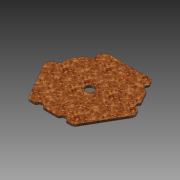
# Autodesk Inventor part: Heatbed_Insulator_Cork
Saved by Autodesk Inventor 2014 (Build 180170000, 170)
## iProperties
Created: 2014-11-03
Part Number: Heatbed_Insulator_Cork
Material: Cork Tiles
Document SubType Name: Modeling
Designer: ThatOtherGuy
Density: 0.11 g/cm^3
Appearance: Cork - Coarse
Author: ThatOtherGuy
Comments: Lowes #34744 or #33530
Autodesk Inventor part; units mm, degrees
ref_plane "YZ Plane" through (0, 0, 0) normal (1, 0, 0) x (0, 1, 0)
ref_plane "XZ Plane" through (0, 0, 0) normal (0, 1, 0) x (-1, 0, 0)
ref_plane "XY Plane" through (0, 0, 0) normal (0, 0, 1) x (1, 0, 0)
sketch "Sketch1" plane through (0, 0, 0) normal (0, 0, 1) x (1, 0, 0)
  line L0 (51.9615, 90) -> (103.923, 0)
  line L1 (103.923, 0) -> (51.9615, -90)
  line L2 (51.9615, -90) -> (-51.9615, -90)
  line L3 (-51.9615, -90) -> (-103.923, 0)
  line L4 (-103.923, 0) -> (-51.9615, 90)
  line L5 (-51.9615, 90) -> (51.9615, 90)
  circle A0 centre (0, 0) radius 10
  dimension "d3" = 180
  dimension "d13" = 20
  constraints: 12 end point, 2 coincident, 1 centre point, 1 horizontal, 13 other
  measures "d3" distance between parallel lines of L2 L5
  measures "d13" diameter of A0
extrude "Extrusion1" add sketch "Sketch1" along normal blind 4.7625
sketch "Sketch2" plane through (0, 0, 0) normal (0, 0, -1) x (-1, 0, 0)
  line L0 (-51.9615, 90) -> (-103.923, 0) projected
  line L1 (51.9615, -90) -> (103.923, 0) projected
  line L2 (103.923, 0) -> (51.9615, 90) projected
  line L3 (51.9615, 90) -> (-51.9615, 90) projected
  line L4 (-51.9615, 90) -> (0, 180) construction
  line L5 (0, 180) -> (51.9615, 90) construction
  arc A0 (-68.5, 61.3545) -> (-61, 74.3449) centre (-64.75, 67.8497) ccw
  arc A1 (-46.6506, 90) -> (-54.617, 85.4006) centre (-46.6506, 80.8013) ccw
  arc A2 (-94.8846, 15.6551) -> (-87.3846, 28.6455) centre (-91.1346, 22.1503) ccw
  line L6 (-103.923, 0) -> (-155.8846, -90) construction
  line L7 (-155.8846, -90) -> (-51.9615, -90) construction
  line L8 (-103.923, 0) -> (-51.9615, -90) projected
  arc A3 (-101.2676, 4.5994) -> (-101.2676, -4.5994) centre (-93.3013, 0) ccw
  point P0 (0, 0)
  dimension "d5" = 7.5
  dimension "d6" = 129.5
  dimension "d7" = 9.1987
  dimension "d8" = 93.3013
  dimension "d9" = 129.5
  constraints: 8 end point, 8 point on circle, 4 centre point, 2 equal radius, 2 parallel, 2 point on line, 2 tangent, 1 collinear, 12 other
  measures "d5" radius of A0
  measures "d6" distance of L4.end A0.centre
  measures "d7" radius of A1
  measures "d8" distance of point (0, 0) A1.centre
  measures "d9" distance of A2.centre L6.end
extrude "Extrusion2" cut sketch "Sketch2" against normal up to next
pattern_circular "Circular Pattern1" count 3 over 360 about axis through (0, 0, 0) along (0, 0, 1) of "Extrusion2"
fillet "Fillet1" radius 5 12 edges at (61, 74.3449, 2.3813) (68.5, 61.3545, 2.3813) (87.3846, 28.6455, 2.3813) (94.8846, 15.6551, 2.3813) (-68.5, 61.3545, 2.3813) (-61, 74.3449, 2.3813) (-94.8846, 15.6551, 2.3813) (-87.3846, 28.6455, 2.3813) (-18.8846, -90, 2.3813) (-33.8846, -90, 2.3813) (33.8846, -90, 2.3813) (18.8846, -90, 2.3813)
equation "\"d9\" = d6"
body "Solid1"
